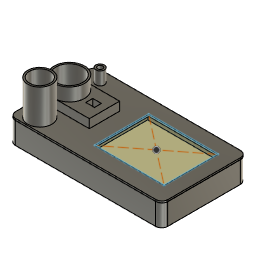
base v5 (Autodesk Fusion 360 design; units mm, degrees)
Autodesk Fusion 360 part; units mm, degrees
sketch "Sketch1" plane through (0, 0, 0) normal (0, 0, 1) x (1, 0, 0)
  line L0 (7, 0) -> (169, 0)
  line L1 (176, 7) -> (176, 91)
  line L2 (169, 98) -> (7, 98)
  line L3 (0, 91) -> (0, 7)
  arc A0 (7, 98) -> (0, 91) centre (7, 91) ccw
  arc A1 (0, 7) -> (7, 0) centre (7, 7) ccw
  arc A2 (176, 91) -> (169, 98) centre (169, 91) ccw
  arc A3 (169, 0) -> (176, 7) centre (169, 7) ccw
  point P0 (176, 0)
  point P1 (0, 98)
  dimension "d1" = 176
  dimension "d2" = 98
  dimension "d3" = 7
  constraint horizontal L0
  constraint vertical L1
  constraint horizontal L2
  constraint vertical L3
  constraint coincident P1 L2
  constraint coincident P1 L3
  constraint tangent L2 A0
  constraint tangent L3 A0
  constraint coincident origin L0
  constraint coincident origin L3
  constraint tangent L0 A1
  constraint tangent L3 A1
  constraint equal A0 A1
  constraint tangent L1 A2
  constraint tangent L2 A2
  constraint equal A0 A2
  constraint coincident P0 L0
  constraint coincident P0 L1
  constraint tangent L0 A3
  constraint tangent L1 A3
  constraint equal A0 A3
  measures "d1" distance of origin P0
  measures "d2" distance of origin P1
  measures "d3" radius of A0
extrude "Extrude1" add sketch "Sketch1" along normal blind 2 makes body 1
extrude "Extrude2" add 1 faces at (115, 32.6667, 2) along direction (0, 0, 1) blind 23 thin wall 1 inside on bodies 1 bodies 1
ref_plane "WorkPlane1" through (88, 49, 17) normal (0, 0, 1) x (1, 0, 0)
sketch "Sketch2" plane through (88, 49, 17) normal (0, 0, 1) x (1, 0, 0)
ref_plane "WorkPlane2" through (88, 49, 25) normal (0, 0, 1) x (1, 0, 0)
sketch "Sketch3" plane through (88, 49, 25) normal (0, 0, 1) x (1, 0, 0)
ref_plane "WorkPlane3" through (88, 49, 25) normal (0, 0, 1) x (1, 0, 0)
sketch "Sketch4" plane through (88, 49, 25) normal (0, 0, 1) x (1, 0, 0)
  line L0 (-80.6728, -48.9627) -> (81.3272, -48.9627)
  line L1 (88.3272, -41.9627) -> (88.3272, 42.0373)
  line L2 (81.3272, 49.0373) -> (-80.6728, 49.0373)
  line L3 (-87.6728, 42.0373) -> (-87.6728, -41.9627)
  arc A0 (-80.6728, 49.0373) -> (-87.6728, 42.0373) centre (-80.6728, 42.0373) ccw
  arc A1 (-87.6728, -41.9627) -> (-80.6728, -48.9627) centre (-80.6728, -41.9627) ccw
  arc A2 (88.3272, 42.0373) -> (81.3272, 49.0373) centre (81.3272, 42.0373) ccw
  arc A3 (81.3272, -48.9627) -> (88.3272, -41.9627) centre (81.3272, -41.9627) ccw
  point P0 (-87.6728, -48.9627)
  point P1 (88.3272, -48.9627)
  point P2 (-87.6728, 49.0373)
  dimension "d13" = 176
  dimension "d14" = 98
  dimension "d15" = 7
  dimension "d16" = 7
  constraint horizontal L0
  constraint vertical L1
  constraint horizontal L2
  constraint vertical L3
  constraint coincident P2 L2
  constraint coincident P2 L3
  constraint tangent L2 A0
  constraint tangent L3 A0
  constraint coincident P0 L0
  constraint coincident P0 L3
  constraint tangent L0 A1
  constraint tangent L3 A1
  constraint equal A0 A1
  constraint tangent L1 A2
  constraint tangent L2 A2
  constraint coincident P1 L0
  constraint coincident P1 L1
  constraint tangent L0 A3
  constraint tangent L1 A3
  constraint equal A2 A3
  measures "d13" distance of P0 P1
  measures "d14" distance of P0 P2
  measures "d15" radius of A0
  measures "d16" radius of A2
extrude "Extrude3" add sketch "Sketch4" along normal blind 2 bodies 1
sketch "Sketch5" plane through (0, 0, 27) normal (0, 0, 1) x (-1, 0, 0)
  arc A0 (-169.3272, -0.0373) -> (-176.3272, -7.0373) centre (-169.3272, -7.0373) ccw
  line L0 (-176.3272, -7.0373) -> (-176.3272, -91.0373)
  arc A1 (-176.3272, -91.0373) -> (-169.3272, -98.0373) centre (-169.3272, -91.0373) ccw
  line L1 (-169.3272, -98.0373) -> (-7.3272, -98.0373)
  arc A2 (-7.3272, -98.0373) -> (-0.3272, -91.0373) centre (-7.3272, -91.0373) ccw
  line L2 (-0.3272, -91.0373) -> (-0.3272, -7.0373)
  arc A3 (-0.3272, -7.0373) -> (-7.3272, -0.0373) centre (-7.3272, -7.0373) ccw
  line L3 (-7.3272, -0.0373) -> (-169.3272, -0.0373)
  circle A4 centre (-19.974, -15.3508) radius 14
  circle A5 centre (-19.974, -15.3508) radius 12
  circle A6 centre (-19.5, -50) radius 17.5
  circle A7 centre (-19.5, -50) radius 15.5
  circle A8 centre (-20, -85) radius 5
  circle A9 centre (-20, -85) radius 3
  line L4 (-19.5, -67.5) -> (-60, -67.5)
  line L5 (-60, -67.5) -> (-60, -32.5)
  line L6 (-60, -32.5) -> (-19.5, -32.5)
  line L7 (-41.75, -54.7442) -> (-51.75, -54.7442)
  line L8 (-51.75, -54.7442) -> (-51.75, -46.7442)
  line L9 (-51.75, -46.7442) -> (-41.75, -46.7442)
  line L10 (-41.75, -46.7442) -> (-41.75, -54.7442)
  dimension "d19" = 28
  dimension "d20" = 24
  dimension "d21" = 35
  dimension "d22" = 31
  dimension "d23" = 10
  dimension "d24" = 6
  dimension "d25" = 10
  dimension "d26" = 8
  constraint concentric A4 A5
  constraint concentric A6 A7
  constraint concentric A8 A9
  constraint coincident A6 L4.start
  constraint tangent A6 L4
  constraint horizontal L4
  constraint perpendicular L4 L5
  constraint coincident A6 L6.end
  constraint tangent A6 L6
  constraint perpendicular L5 L6
  constraint horizontal L7
  constraint vertical L8
  constraint horizontal L9
  constraint vertical L10
  measures "d19" diameter of A4
  measures "d20" diameter of A5
  measures "d21" diameter of A6
  measures "d22" diameter of A7
  measures "d23" diameter of A8
  measures "d24" diameter of A9
  measures "d25" distance of L7.start L7.end
  measures "d26" distance of L7.start L9.end
extrude "Extrude4" add sketch "Sketch5" along normal blind 25 contours A6 bodies 1
extrude "Extrude5" add sketch "Sketch5" along normal blind 40 contours A4 bodies 1
extrude "Extrude6" add sketch "Sketch5" along normal blind 10 contours A6 L4 L5 L6 bodies 1
extrude "Extrude7" add sketch "Sketch5" along normal blind 15 contours A8 bodies 1
sketch "Sketch7" plane through (0, 0, 27) normal (0, 0, 1) x (1, 0, 0)
sketch "Sketch8" plane through (0, 0, 27) normal (0, 0, 1) x (-1, 0, 0)
  line L0 (-80, -81.11) -> (-160, -81.11)
  line L1 (-160, -81.11) -> (-160, -18.89)
  line L2 (-160, -18.89) -> (-80, -18.89)
  line L3 (-80, -18.89) -> (-80, -81.11)
  line L4 (-80, -81.11) -> (-160, -18.89) construction
  line L5 (-160, -81.11) -> (-80, -18.89) construction
  point P0 (-120, -50)
  dimension "d38" = 80
  dimension "d39" = 62.22
  constraint horizontal L0
  constraint perpendicular L0 L1
  constraint parallel L0 L2
  constraint parallel L1 L3
  constraint coincident L4 P0
  constraint coincident L5 P0
  measures "d38" distance of L1.end L2.end
  measures "d39" distance of L0.end L1.end
ref_plane "WorkPlane4" through (0, 0, 0) normal (0, 1, 0) x (0, 0, 1)
ref_plane "WorkPlane5" through (120, 50, 17) normal (0, 0, 1) x (-1, 0, 0)
sketch "Sketch9" plane through (88, 49, 17) normal (0, 0, 1) x (1, 0, 0)
  line L0 (76.8954, -33.9188) -> (-13.1046, -33.9188)
  line L1 (-13.1046, -33.9188) -> (-13.1046, 36.0812)
  line L2 (-13.1046, 36.0812) -> (76.8954, 36.0812)
  line L3 (76.8954, 36.0812) -> (76.8954, -33.9188)
  line L4 (76.8954, -33.9188) -> (-13.1046, 36.0812) construction
  line L5 (-13.1046, -33.9188) -> (76.8954, 36.0812) construction
  point P0 (31.8954, 1.0812)
  dimension "d42" = 90
  dimension "d43" = 70
  constraint horizontal L0
  constraint perpendicular L0 L1
  constraint parallel L0 L2
  constraint parallel L1 L3
  constraint coincident L4 P0
  constraint coincident L5 P0
  measures "d42" distance of L1.end L2.end
  measures "d43" distance of L0.end L1.end
loft "Loft1" add profiles "Sketch9", "Sketch8" section 1 section 2 separate body makes body 2
surface "Extrude8" add extruded along (0, 0, 1) between 0 and -2 1 faces at (106.6667, 60.37, 27) separate body on bodies 2 makes body 3
delete_face "SurfaceDeleteFace1" leaving the opening 1 faces at (106.6667, 60.37, 27) on bodies 2
extrude "Extrude9" cut sketch "Sketch8" against normal blind 12 bodies 1
sketch "Sketch10" plane through (88, 49, 25) normal (0, 0, 1) x (1, 0, 0)
